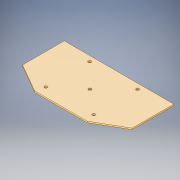
# Autodesk Inventor part: DPLX_P022 Spark Gap Shielding Top
Saved by Autodesk Inventor 2018 (Build 220112000, 112)
## iProperties
Created: 2017-11-28
Part Number: DPLX_P022 Spark Gap Shielding Top
Material: Polyethylene, High Density
Document SubType Name: Modeling
Designer: Sam
Density: 0.952 g/cm^3
Appearance: Smooth - Off-White
Mass: 11.4244 g
Surface Area: 163.799 cm^2
Volume: 12.0005 cm^3
Author: Sam
Comments: http://www.eplastics.com/Plastic/G9-G10-FR4-glass-epoxy-sheet/G10NAT-060X12X12
Autodesk Inventor part; units mm, degrees
ref_plane "YZ Plane" through (0, 0, 0) normal (1, 0, 0) x (0, 1, 0)
ref_plane "XZ Plane" through (0, 0, 0) normal (0, 1, 0) x (-1, 0, 0)
ref_plane "XY Plane" through (0, 0, 0) normal (0, 0, 1) x (1, 0, 0)
sketch "Sketch1" plane through (0, 0, 0) normal (0, 1, 0) x (-1, 0, 0)
  line L0 (-63.5, 33.655) -> (63.5, 33.655)
  line L1 (63.5, 33.655) -> (63.5, -33.655)
  line L2 (63.5, -33.655) -> (-63.5, -33.655)
  line L3 (-63.5, -33.655) -> (-63.5, 33.655)
  line L4 (-63.5, 33.655) -> (63.5, -33.655) construction
  line L5 (63.5, 33.655) -> (-63.5, -33.655) construction
  point P0 (0, 0)
  dimension "d0" = 127
  dimension "d1" = 67.31
  constraints: 12 end point, 2 midpoint, 2 parallel, 1 horizontal, 1 perpendicular
  measures "d0" distance of L1.end L2.end
  measures "d1" distance of L0.end L1.end
extrude "Extrusion1" add sketch "Sketch1" along normal mid plane 1.524
chamfer "Chamfer1" distance 19.05 angle 60 1 edges at (-63.5, 0, 33.655) measured on face at (-63.5, -0.254, 11.2183)
sketch "Sketch3" plane through (0, 0.762, 0) normal (0, 1, 0) x (1, 0, 0)
  circle A0 centre (27.7749, 27.4042) radius 1.7018 projected
  circle A1 centre (27.7749, -23.3958) radius 1.7018 projected
  circle A2 centre (-27.7751, -23.3958) radius 1.7018 projected
  circle A3 centre (-27.7751, 27.4042) radius 1.7018 projected
  point P0 (0, 0)
hole "Hole2" at (0, 0.762, 0) at (27.7749, 0.762, -27.4042) at (27.7749, 0.762, 23.3958) at (-27.7751, 0.762, 23.3958) at (-27.7751, 0.762, -27.4042) direction (0, -1, 0) diameter 3.4036 end through all clearance for "Flat Head Machine Screw" size "M3" standard "Ansi Metric M Profile"
chamfer "Chamfer2" distance 19.05 angle 60 1 edges at (63.5, 0, 33.655) measured on face at (63.5, 0.254, 11.2183)
body "Solid1"
